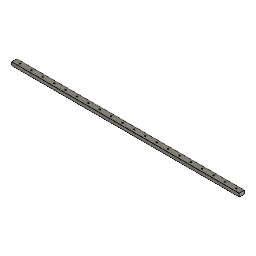
_Linear Rail Mock.78ead6d0-6ba2-4e63-ae19-307b231ec727 (Autodesk Fusion 360 design; units mm, degrees)
Autodesk Fusion 360 part; units mm, degrees
sketch "Sketch1" plane through (0, 0, 0) normal (1, 0, 0) x (0, 1, 0)
  line L0 (0.5, 0) -> (11.5, 0)
  line L1 (12, 0.5) -> (12, 7.5)
  line L2 (11.5, 8) -> (0.5, 8)
  line L3 (0, 7.5) -> (0, 0.5)
  line L4 (0, 0) -> (0, 0.3672)
  line L5 (0, 0) -> (0, 5)
  arc A0 (11.5, 0) -> (12, 0.5) centre (11.5, 0.5) ccw
  arc A1 (0, 0.5) -> (0.5, 0) centre (0.5, 0.5) ccw
  line L6 (12, 7.5) -> (11.5, 7.5)
  line L7 (11.5, 7.5) -> (11.5, 8)
  line L8 (11.5, 8) -> (12, 8)
  line L9 (12, 8) -> (12, 7.5)
  line L10 (0.5, 8) -> (0, 8)
  line L11 (0, 8) -> (0, 7.5)
  line L12 (0, 7.5) -> (0.5, 7.5)
  line L13 (0.5, 7.5) -> (0.5, 8)
  dimension "d1" = 12
  dimension "d2" = 8
  measures "d1" distance of L4.start
  measures "d2" distance of L4.start
extrude "Extrude1" add sketch "Sketch1" along normal blind 500
sketch "Sketch2" plane through (0, 0, 8) normal (0, 0, 1) x (-1, 0, 0)
  line L0 (0, -12) -> (0, 0)
  line L1 (-500, 0) -> (-500, -12)
  circle A0 centre (-488, -6) radius 1.5
  circle A1 centre (-463, -6) radius 1.5
  circle A2 centre (-438, -6) radius 1.5
  circle A3 centre (-413, -6) radius 1.5
  circle A4 centre (-388, -6) radius 1.5
  circle A5 centre (-363, -6) radius 1.5
  circle A6 centre (-338, -6) radius 1.5
  circle A7 centre (-313, -6) radius 1.5
  circle A8 centre (-288, -6) radius 1.5
  circle A9 centre (-263, -6) radius 1.5
  circle A10 centre (-238, -6) radius 1.5
  circle A11 centre (-213, -6) radius 1.5
  circle A12 centre (-188, -6) radius 1.5
  circle A13 centre (-163, -6) radius 1.5
  circle A14 centre (-138, -6) radius 1.5
  circle A15 centre (-113, -6) radius 1.5
  circle A16 centre (-88, -6) radius 1.5
  circle A17 centre (-63, -6) radius 1.5
  circle A18 centre (-38, -6) radius 1.5
  circle A19 centre (-13, -6) radius 1.5
  line L2 (0, 0) -> (-500, 0)
  line L3 (-500, -12) -> (0, -12)
  dimension "d6" = 3
  dimension "d7" = 12
  dimension "d10" = 25
  dimension "d11" = 0
  measures "d6" diameter of A0
  measures "d7" distance of L1
extrude "Extrude2" cut sketch "Sketch2" against normal blind 50 contours A0 | A1 | A2 | A3 | A4 | A5 | A6 | A7 | A8 | A9 | A10 | A11 | A12 | A13 | A14 | A15 | A16 | A17 | A18 | A19
